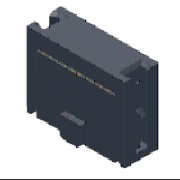
# Autodesk Inventor part: RC CON_16CKT
Saved by Autodesk Inventor 2017 (Build 210142000, 142)
## iProperties
Created: 2016-02-22
Part Number: RC CON_16CKT
Material: Générique
Description: 2,54 mm (0,10 po) Pas, Prise, Vertical, Double ligne
Document SubType Name: Modeling
Designer: Adrien MARY
Language: fr-FR
Size Designation: Ribbon Cable Connector-04
Categories: <MemberInstance><Categories><Category DisplayName="Câble et faisceau" InternalName="e4a7e005-5e42-4d16-b293-125e7f0d0512" Mnemonic="CABLEANDHARNESS"><Category DisplayName="Raccords" InternalName="6f634eba-a678-4820-a31d-2c2d5ee6728e" Mnemonic="CONNECTORS"><CategoryParameter DisplayName="RefDes" InternalName="c3740e8c-60ab-4d5d-8584-52b73222f2f0" Mnemonic="REFDES"/><Category DisplayName="Câble-ruban" InternalName="27621a3d-53ec-49ed-8225-e2ac65e8eb52" Mnemonic="RIBBONCABLE"/></Category></Category><Category DisplayName="Type de données" InternalName="23b78d0f-2648-40c6-8793-ca6db495c9e8" Mnemonic="DATATYPE"><CategoryParameter DisplayName="AfficherNom" InternalName="05415f3d-3907-474b-a020-eb9d644f4cf3" Mnemonic="DISPLAYNAME"/><CategoryParameter DisplayName="Norme" InternalName="0c0a119c-1e12-4c84-803f-101930972f5e" Mnemonic="STANDARD"/><CategoryParameter DisplayName="Description" InternalName="13903e3d-64b1-4950-80da-f627842ea37f" Mnemonic="DESCRIPTION"/><CategoryParameter DisplayName="Désignation" InternalName="2675968c-4ce5-49e0-a4f5-552d29089031" Mnemonic="DESIGNATION"/><CategoryParameter DisplayName="Ligne par défaut" InternalName="2af9ec52-faaa-4026-b378-f9fa4afca842" Mnemonic="DEFAULTROW"/><CategoryParameter DisplayName="Nom de dossier" InternalName="3f06958e-8713-4116-9be7-ed6184ecc97b" Mnemonic="FOLDERNAME"/><CategoryParameter DisplayName="Guide révision" InternalName="45a75005-10b1-4dfc-8d6d-dfe629f0b93c" Mnemonic="REVISIONGUID"/><CategoryParameter DisplayName="NomFichier" InternalName="8b46a4cc-9585-4fed-90c3-899f57e09a73" Mnemonic="FILENAME"/><CategoryParameter DisplayName="OrgNorm" InternalName="8f5914e1-4693-403f-8ab5-d37768198c9d" Mnemonic="STDSORG"/><CategoryParameter DisplayName="Version de la famille" InternalName="914462f6-6e19-4b14-ba84-155b9680b1d0" Mnemonic="FAMILYREVISION"/><CategoryParameter DisplayName="Version standard" InternalName="91d5a463-65c2-4fde-b823-3b7fea5e8e17" Mnemonic="STANDARDREVISION"/><CategoryParameter DisplayName="Révision de membre" InternalName="a65d44b9-392f-4f4f-857b-e4b3d54996fe" Mnemonic="MEMBERREVISION"/><CategoryParameter DisplayName="DélimiterFormat" InternalName="bc51e27b-3422-4e78-93ef-cec197ddf230" Mnemonic="CLIPFORMAT"/><CategoryParameter DisplayName="Fabricant" InternalName="cd6c7a72-a28a-4e50-99a9-2c7f4e13e5ad" Mnemonic="MANUFACTURER"/><CategoryParameter DisplayName="NomInterne" InternalName="cf1d0246-76d9-4b4a-8305-fa0409afb5c1" Mnemonic="INTERNALNAME"/><CategoryParameter DisplayName="Métrique" InternalName="e2385c5b-1ea4-4823-96a8-8de651266ec3" Mnemonic="ISMETRIC"/><Category DisplayName="Pièce" InternalName="c0e0b642-3bcb-4cc8-9e80-f96d35c4afa4" Mnemonic="PART"><CategoryParameter DisplayName="Numéro de pièce" InternalName="016b6077-bfbe-49bd-92c9-d8d59c39c941" Mnemonic="PARTNUMBER"/><CategoryParameter DisplayName="Numéro de stock" InternalName="4dba7c1c-e26c-444e-836c-b08b433409a8" Mnemonic="STOCKNUMBER"/><CategoryParameter DisplayName="Clé matière" InternalName="5c9a8adb-dd2b-4535-b97f-0a94a95fe41f" Mnemonic="MATERIALKEY"/><CategoryParameter DisplayName="Matière" InternalName="818a152a-d3c3-49ca-80ee-df7d91421b8e" Mnemonic="MATERIAL"/></Category></Category></Categories><FamilyTemplate Id="Ribbon Cable Connector"><FamilyTemplateParameters><FamilyTemplateParameter ObjectType="kUserParameterObject" ValueType="xs:double" Id="1" ObjectReferenceKey="Circuits"/><FamilyTemplateParameter ObjectType="kUserParameterObject" ValueType="xs:double" Id="2" ObjectReferenceKey="DimA"/><FamilyTemplateParameter ObjectType="kUserParameterObject" ValueType="xs:double" Id="3" ObjectReferenceKey="DimB"/><FamilyTemplateParameter ObjectType="kPropertyObject" ValueType="xs:string" Id="100" ObjectReferenceKey="{32853F0F-3444-11d1-9E93-0060B03C1CA6}" SubObjectId="52"/><FamilyTemplateParameter ObjectType="kPropertyObject" ValueType="xs:string" Id="105" ObjectReferenceKey="{32853F0F-3444-11d1-9E93-0060B03C1CA6}" SubObjectId="5"/><FamilyTemplateParameter ObjectType="kPartComponentDefinitionObject" ValueType="xs:string" Id="110" SubObjectId="Material"/><FamilyTemplateParameter ObjectType="kPartFeatureObject" ValueType="xs:boolean" Id="200" ObjectReferenceKey="1002000010000000700a0100000000008000000000000000" SubObjectId="Suppressed"/><FamilyTemplateParameter ObjectType="kPartFeatureObject" ValueType="xs:boolean" Id="201" ObjectReferenceKey="1002000010000000320b0100000000008000000000000000" SubObjectId="Suppressed"/><FamilyTemplateParameter ObjectType="kPartFeatureObject" ValueType="xs:boolean" Id="202" ObjectReferenceKey="100200001000000044680200000000008000000000000000" SubObjectId="Suppressed"/><FamilyTemplateParameter ObjectType="kPartFeatureObject" ValueType="xs:boolean" Id="203" ObjectReferenceKey="100200001000000061680200000000008000000000000000" SubObjectId="Suppressed"/><FamilyTemplateParameter ObjectType="kPartFeatureObject" ValueType="xs:boolean" Id="204" ObjectReferenceKey="100200001000000064680200000000008000000000000000" SubObjectId="Suppressed"/><FamilyTemplateParameter ObjectType="kPartFeatureObject" ValueType="xs:boolean" Id="205" ObjectReferenceKey="100200001000000067680200000000008000000000000000" SubObjectId="Suppressed"/><FamilyTemplateParameter ObjectType="kPartFeatureObject" ValueType="xs:boolean" Id="206" ObjectReferenceKey="10020000100000006a680200000000008000000000000000" SubObjectId="Suppressed"/><FamilyTemplateParameter ObjectType="kPartFeatureObject" ValueType="xs:boolean" Id="207" ObjectReferenceKey="10020000100000006d680200000000008000000000000000" SubObjectId="Suppressed"/><FamilyTemplateParameter ObjectType="kPartFeatureObject" ValueType="xs:boolean" Id="208" ObjectReferenceKey="100200001000000070680200000000008000000000000000" SubObjectId="Suppressed"/><FamilyTemplateParameter ObjectType="kPartFeatureObject" ValueType="xs:boolean" Id="209" ObjectReferenceKey="100200001000000073680200000000008000000000000000" SubObjectId="Suppressed"/><FamilyTemplateParameter ObjectType="kPartFeatureObject" ValueType="xs:boolean" Id="210" ObjectReferenceKey="100200001000000076680200000000008000000000000000" SubObjectId="Suppressed"/><FamilyTemplateParameter ObjectType="kPartFeatureObject" ValueType="xs:boolean" Id="211" ObjectReferenceKey="100200001000000079680200000000008000000000000000" SubObjectId="Suppressed"/><FamilyTemplateParameter ObjectType="kPartFeatureObject" ValueType="xs:boolean" Id="212" ObjectReferenceKey="10020000100000007c680200000000008000000000000000" SubObjectId="Suppressed"/><FamilyTemplateParameter ObjectType="kPartFeatureObject" ValueType="xs:boolean" Id="213" ObjectReferenceKey="100200001000000047680200000000008000000000000000" SubObjectId="Suppressed"/><FamilyTemplateParameter ObjectType="kPartFeatureObject" ValueType="xs:boolean" Id="214" ObjectReferenceKey="10020000100000007f680200000000008000000000000000" SubObjectId="Suppressed"/><FamilyTemplateParameter ObjectType="kPartFeatureObject" ValueType="xs:boolean" Id="215" ObjectReferenceKey="100200001000000082680200000000008000000000000000" SubObjectId="Suppressed"/><FamilyTemplateParameter ObjectType="kPartFeatureObject" ValueType="xs:boolean" Id="216" ObjectReferenceKey="100200001000000085680200000000008000000000000000" SubObjectId="Suppressed"/><FamilyTemplateParameter ObjectType="kPartFeatureObject" ValueType="xs:boolean" Id="217" ObjectReferenceKey="100200001000000088680200000000008000000000000000" SubObjectId="Suppressed"/><FamilyTemplateParameter ObjectType="kPartFeatureObject" ValueType="xs:boolean" Id="218" ObjectReferenceKey="10020000100000008b680200000000008000000000000000" SubObjectId="Suppressed"/><FamilyTemplateParameter ObjectType="kPartFeatureObject" ValueType="xs:boolean" Id="219" ObjectReferenceKey="10020000100000008e680200000000008000000000000000" SubObjectId="Suppressed"/><FamilyTemplateParameter ObjectType="kPartFeatureObject" ValueType="xs:boolean" Id="220" ObjectReferenceKey="100200001000000091680200000000008000000000000000" SubObjectId="Suppressed"/><FamilyTemplateParameter ObjectType="kPartFeatureObject" ValueType="xs:boolean" Id="221" ObjectReferenceKey="100200001000000094680200000000008000000000000000" SubObjectId="Suppressed"/><FamilyTemplateParameter ObjectType="kPartFeatureObject" ValueType="xs:boolean" Id="222" ObjectReferenceKey="100200001000000097680200000000008000000000000000" SubObjectId="Suppressed"/><FamilyTemplateParameter ObjectType="kPartFeatureObject" ValueType="xs:boolean" Id="223" ObjectReferenceKey="10020000100000009a680200000000008000000000000000" SubObjectId="Suppressed"/><FamilyTemplateParameter ObjectType="kPartFeatureObject" ValueType="xs:boolean" Id="224" ObjectReferenceKey="10020000100000004a680200000000008000000000000000" SubObjectId="Suppressed"/><FamilyTemplateParameter ObjectType="kPartFeatureObject" ValueType="xs:boolean" Id="225" ObjectReferenceKey="10020000100000009d680200000000008000000000000000" SubObjectId="Suppressed"/><FamilyTemplateParameter ObjectType="kPartFeatureObject" ValueType="xs:boolean" Id="226" ObjectReferenceKey="1002000010000000a0680200000000008000000000000000" SubObjectId="Suppressed"/><FamilyTemplateParameter ObjectType="kPartFeatureObject" ValueType="xs:boolean" Id="227" ObjectReferenceKey="1002000010000000a3680200000000008000000000000000" SubObjectId="Suppressed"/><FamilyTemplateParameter ObjectType="kPartFeatureObject" ValueType="xs:boolean" Id="228" ObjectReferenceKey="1002000010000000a6680200000000008000000000000000" SubObjectId="Suppressed"/><FamilyTemplateParameter ObjectType="kPartFeatureObject" ValueType="xs:boolean" Id="229" ObjectReferenceKey="1002000010000000a9680200000000008000000000000000" SubObjectId="Suppressed"/><FamilyTemplateParameter ObjectType="kPartFeatureObject" ValueType="xs:boolean" Id="230" ObjectReferenceKey="1002000010000000ac680200000000008000000000000000" SubObjectId="Suppressed"/><FamilyTemplateParameter ObjectType="kPartFeatureObject" ValueType="xs:boolean" Id="231" ObjectReferenceKey="1002000010000000af680200000000008000000000000000" SubObjectId="Suppressed"/><FamilyTemplateParameter ObjectType="kPartFeatureObject" ValueType="xs:boolean" Id="232" ObjectReferenceKey="1002000010000000b2680200000000008000000000000000" SubObjectId="Suppressed"/><FamilyTemplateParameter ObjectType="kPartFeatureObject" ValueType="xs:boolean" Id="233" ObjectReferenceKey="1002000010000000b5680200000000008000000000000000" SubObjectId="Suppressed"/><FamilyTemplateParameter ObjectType="kPartFeatureObject" ValueType="xs:boolean" Id="234" ObjectReferenceKey="1002000010000000b8680200000000008000000000000000" SubObjectId="Suppressed"/><FamilyTemplateParameter ObjectType="kPartFeatureObject" ValueType="xs:boolean" Id="235" ObjectReferenceKey="10020000100000004f680200000000008000000000000000" SubObjectId="Suppressed"/><FamilyTemplateParameter ObjectType="kPartFeatureObject" ValueType="xs:boolean" Id="236" ObjectReferenceKey="1002000010000000bb680200000000008000000000000000" SubObjectId="Suppressed"/><FamilyTemplateParameter ObjectType="kPartFeatureObject" ValueType="xs:boolean" Id="237" ObjectReferenceKey="1002000010000000be680200000000008000000000000000" SubObjectId="Suppressed"/><FamilyTemplateParameter ObjectType="kPartFeatureObject" ValueType="xs:boolean" Id="238" ObjectReferenceKey="1002000010000000c1680200000000008000000000000000" SubObjectId="Suppressed"/><FamilyTemplateParameter ObjectType="kPartFeatureObject" ValueType="xs:boolean" Id="239" ObjectReferenceKey="1002000010000000c4680200000000008000000000000000" SubObjectId="Suppressed"/><FamilyTemplateParameter ObjectType="kPartFeatureObject" ValueType="xs:boolean" Id="240" ObjectReferenceKey="1002000010000000c7680200000000008000000000000000" SubObjectId="Suppressed"/><FamilyTemplateParameter ObjectType="kPartFeatureObject" ValueType="xs:boolean" Id="241" ObjectReferenceKey="1002000010000000ca680200000000008000000000000000" SubObjectId="Suppressed"/><FamilyTemplateParameter ObjectType="kPartFeatureObject" ValueType="xs:boolean" Id="242" ObjectReferenceKey="1002000010000000cd680200000000008000000000000000" SubObjectId="Suppressed"/><FamilyTemplateParameter ObjectType="kPartFeatureObject" ValueType="xs:boolean" Id="243" ObjectReferenceKey="1002000010000000d0680200000000008000000000000000" SubObjectId="Suppressed"/><FamilyTemplateParameter ObjectType="kPartFeatureObject" ValueType="xs:boolean" Id="244" ObjectReferenceKey="1002000010000000d3680200000000008000000000000000" SubObjectId="Suppressed"/><FamilyTemplateParameter ObjectType="kPartFeatureObject" ValueType="xs:boolean" Id="245" ObjectReferenceKey="1002000010000000d6680200000000008000000000000000" SubObjectId="Suppressed"/><FamilyTemplateParameter ObjectType="kPartFeatureObject" ValueType="xs:boolean" Id="246" ObjectReferenceKey="100200001000000052680200000000008000000000000000" SubObjectId="Suppressed"/><FamilyTemplateParameter ObjectType="kPartFeatureObject" ValueType="xs:boolean" Id="247" ObjectReferenceKey="1002000010000000d9680200000000008000000000000000" SubObjectId="Suppressed"/><FamilyTemplateParameter ObjectType="kPartFeatureObject" ValueType="xs:boolean" Id="248" ObjectReferenceKey="1002000010000000dc680200000000008000000000000000" SubObjectId="Suppressed"/><FamilyTemplateParameter ObjectType="kPartFeatureObject" ValueType="xs:boolean" Id="249" ObjectReferenceKey="1002000010000000df680200000000008000000000000000" SubObjectId="Suppressed"/><FamilyTemplateParameter ObjectType="kPartFeatureObject" ValueType="xs:boolean" Id="250" ObjectReferenceKey="1002000010000000e2680200000000008000000000000000" SubObjectId="Suppressed"/><FamilyTemplateParameter ObjectType="kPartFeatureObject" ValueType="xs:boolean" Id="251" ObjectReferenceKey="1002000010000000e5680200000000008000000000000000" SubObjectId="Suppressed"/><FamilyTemplateParameter ObjectType="kPartFeatureObject" ValueType="xs:boolean" Id="252" ObjectReferenceKey="1002000010000000e8680200000000008000000000000000" SubObjectId="Suppressed"/><FamilyTemplateParameter ObjectType="kPartFeatureObject" ValueType="xs:boolean" Id="253" ObjectReferenceKey="1002000010000000eb680200000000008000000000000000" SubObjectId="Suppressed"/><FamilyTemplateParameter ObjectType="kPartFeatureObject" ValueType="xs:boolean" Id="254" ObjectReferenceKey="1002000010000000ee680200000000008000000000000000" SubObjectId="Suppressed"/><FamilyTemplateParameter ObjectType="kPartFeatureObject" ValueType="xs:boolean" Id="255" ObjectReferenceKey="1002000010000000f1680200000000008000000000000000" SubObjectId="Suppressed"/><FamilyTemplateParameter ObjectType="kPartFeatureObject" ValueType="xs:boolean" Id="256" ObjectReferenceKey="1002000010000000f4680200000000008000000000000000" SubObjectId="Suppressed"/><FamilyTemplateParameter ObjectType="kPartFeatureObject" ValueType="xs:boolean" Id="257" ObjectReferenceKey="100200001000000055680200000000008000000000000000" SubObjectId="Suppressed"/><FamilyTemplateParameter ObjectType="kPartFeatureObject" ValueType="xs:boolean" Id="258" ObjectReferenceKey="1002000010000000f7680200000000008000000000000000" SubObjectId="Suppressed"/><FamilyTemplateParameter ObjectType="kPartFeatureObject" ValueType="xs:boolean" Id="259" ObjectReferenceKey="1002000010000000fa680200000000008000000000000000" SubObjectId="Suppressed"/><FamilyTemplateParameter ObjectType="kPartFeatureObject" ValueType="xs:boolean" Id="260" ObjectReferenceKey="1002000010000000fd680200000000008000000000000000" SubObjectId="Suppressed"/><FamilyTemplateParameter ObjectType="kPartFeatureObject" ValueType="xs:boolean" Id="261" ObjectReferenceKey="100200001000000000690200000000008000000000000000" SubObjectId="Suppressed"/><FamilyTemplateParameter ObjectType="kPartFeatureObject" ValueType="xs:boolean" Id="262" ObjectReferenceKey="100200001000000003690200000000008000000000000000" SubObjectId="Suppressed"/><FamilyTemplateParameter ObjectType="kPartFeatureObject" ValueType="xs:boolean" Id="263" ObjectReferenceKey="100200001000000058680200000000008000000000000000" SubObjectId="Suppressed"/><FamilyTemplateParameter ObjectType="kPartFeatureObject" ValueType="xs:boolean" Id="264" ObjectReferenceKey="10020000100000005b680200000000008000000000000000" SubObjectId="Suppressed"/><FamilyTemplateParameter ObjectType="kPartFeatureObject" ValueType="xs:boolean" Id="265" ObjectReferenceKey="10020000100000005e680200000000008000000000000000" SubObjectId="Suppressed"/></FamilyTemplateParameters></FamilyTemplate><CategoryParameterMap><ParamToTemplateMap><ParamToTemplate CategoryParameter="//CategoryParameter[@InternalName='05415f3d-3907-474b-a020-eb9d644f4cf3']" ConstantValue="Ribbon Cable Connector"/><ParamToTemplate CategoryParameter="//CategoryParameter[@InternalName='0c0a119c-1e12-4c84-803f-101930972f5e']" TemplateParameter="102"/><ParamToTemplate CategoryParameter="//CategoryParameter[@InternalName='13903e3d-64b1-4950-80da-f627842ea37f']" ConstantValue="2.54mm (0.10in) Pitch, Receptacle, Vertical, Dual Row"/><ParamToTemplate CategoryParameter="//CategoryParameter[@InternalName='2af9ec52-faaa-4026-b378-f9fa4afca842']" ConstantValue="1"/><ParamToTemplate CategoryParameter="//CategoryParameter[@InternalName='3f06958e-8713-4116-9be7-ed6184ecc97b']" ConstantValue="Ribbon Cable Connector"/><ParamToTemplate CategoryParameter="//CategoryParameter[@InternalName='45a75005-10b1-4dfc-8d6d-dfe629f0b93c']" ConstantValue="a3a57e36-970e-4b53-b58b-44e930e7e04d"/><ParamToTemplate CategoryParameter="//CategoryParameter[@InternalName='8f5914e1-4693-403f-8ab5-d37768198c9d']" TemplateParameter="101"/><ParamToTemplate CategoryParameter="//CategoryParameter[@InternalName='914462f6-6e19-4b14-ba84-155b9680b1d0']" ConstantValue="11"/><ParamToTemplate CategoryParameter="//CategoryParameter[@InternalName='91d5a463-65c2-4fde-b823-3b7fea5e8e17']" TemplateParameter="103"/><ParamToTemplate CategoryParameter="//CategoryParameter[@InternalName='bc51e27b-3422-4e78-93ef-cec197ddf230']" ConstantValue="CF_INVENTOR.STDPARTS"/><ParamToTemplate CategoryParameter="//CategoryParameter[@InternalName='cd6c7a72-a28a-4e50-99a9-2c7f4e13e5ad']" TemplateParameter="104"/><ParamToTemplate CategoryParameter="//CategoryParameter[@InternalName='cf1d0246-76d9-4b4a-8305-fa0409afb5c1']" ConstantValue="40b76d18-17cd-4eeb-a7c8-2b6dc5bd681a"/><ParamToTemplate CategoryParameter="//CategoryParameter[@InternalName='e2385c5b-1ea4-4823-96a8-8de651266ec3']" ConstantValue="true"/><ParamToTemplate CategoryParameter="//CategoryParameter[@InternalName='8b46a4cc-9585-4fed-90c3-899f57e09a73']" ConstantValue="Ribbon Cable Connector-04"/><ParamToTemplate CategoryParameter="//CategoryParameter[@InternalName='a65d44b9-392f-4f4f-857b-e4b3d54996fe']" ConstantValue="b666cb32-0b43-4429-87d9-31e43f82d377"/><ParamToTemplate CategoryParameter="//CategoryParameter[@InternalName='2675968c-4ce5-49e0-a4f5-552d29089031']" TemplateParameter="100"/><ParamToTemplate CategoryParameter="//CategoryParameter[@InternalName='818a152a-d3c3-49ca-80ee-df7d91421b8e']" TemplateParameter="110"/><ParamToTemplate CategoryParameter="//CategoryParameter[@InternalName='016b6077-bfbe-49bd-92c9-d8d59c39c941']" TemplateParameter="105"/></ParamToTemplateMap></CategoryParameterMap></MemberInstance>
Density: 1 g/cm^3
Appearance: Dark Gray
IsCustomPart: 0
Author: Adrien MARY
Autodesk Inventor part; units mm, degrees
ref_plane "YZ Plane" through (0, 0, 0) normal (1, 0, 0) x (0, 1, 0)
ref_plane "XZ Plane" through (0, 0, 0) normal (0, 1, 0) x (-1, 0, 0)
ref_plane "XY Plane" through (0, 0, 0) normal (0, 0, 1) x (1, 0, 0)
sketch "Sketch1" plane through (0, 0, 0) normal (0, 0, 1) x (1, 0, 0)
  line L0 (10.79, -3) -> (-10.79, -3)
  line L1 (-10.79, -1.5) -> (-10.04, -1.5)
  line L2 (-10.04, -1.5) -> (-10.04, -2.1)
  line L3 (-10.04, -2.1) -> (-10.79, -2.1)
  line L4 (-10.79, -3) -> (-10.79, -2.1)
  line L5 (-10.79, -1.5) -> (-10.79, 3)
  line L6 (10.04, 2.1) -> (10.79, 2.1)
  line L7 (10.79, 1.5) -> (10.04, 1.5)
  line L8 (10.04, 1.5) -> (10.04, 2.1)
  line L9 (10.79, 3) -> (10.79, 2.1)
  line L10 (10.79, 1.5) -> (10.79, -3)
  line L11 (0, 3) -> (0, -3) construction
  line L12 (-10.79, 3) -> (10.79, 3)
  point P0 (0, 0)
  point P1 (0, 0)
  dimension "d0" = 21.58
  dimension "d1" = 6
  dimension "d4" = 0.9
  dimension "d5" = 0.75
  dimension "d6" = 0.6
  dimension "d8" = 0.75
  dimension "d9" = 0.6
  dimension "d10" = 6
  dimension "d12" = 0.9
  constraints: 26 end point, 8 parallel, 3 midpoint, 3 perpendicular, 2 horizontal, 1 coincident
  measures "d0" distance of L0.start L0.end
  measures "d1" distance of L0.end L5.end
  measures "d4" distance between parallel lines of L0 L3
  measures "d5" distance of L2.end L4.end
  measures "d6" distance of L2.start L2.end
  measures "d8" distance of L8.end L6.end
  measures "d9" distance of L8.start L8.end
  measures "d10" distance of L0.start L9.start
  measures "d12" distance of L9.start L6.end
extrude "Extrusion1" add sketch "Sketch1" along normal blind 10.2
sketch "Sketch2" plane through (-10.79, -3, 0) normal (0, -1, 0) x (1, 0, 0)
  line L0 (0, 0) -> (21.58, 0) projected
  line L1 (8.99, 3.6) -> (12.59, 3.6)
  line L2 (12.59, 3.6) -> (12.59, 0.5)
  line L3 (12.09, 0) -> (9.49, 0)
  line L4 (8.99, 0.5) -> (8.99, 3.6)
  line L5 (8.99, 0.5) -> (9.49, 0)
  line L6 (12.59, 0.5) -> (12.09, 0)
  point P0 (10.79, 0)
  dimension "d15" = 3.6
  dimension "d17" = 0.5
  dimension "d19" = 135
  dimension "d20" = 135
  dimension "d21" = 0.5
  dimension "d22" = 3.6
  constraints: 12 end point, 2 midpoint, 2 parallel, 1 horizontal, 1 perpendicular
  measures "d15" distance of L1.start L1.end
  measures "d17" horizontal distance of L3.end L4.start
  measures "d19" angle of L5 L4
  measures "d20" angle of L6 L2
  measures "d21" horizontal distance of L3.start L2.end
  measures "d22" distance between parallel lines of L0 L1
extrude "Extrusion2" add sketch "Sketch2" along normal blind 1
sketch "Sketch3" plane through (0, 0, 0) normal (0, 1, 0) x (-1, 0, 0)
  line L0 (-10.79, 3.6) -> (-11.04, 3.6)
  line L1 (-11.79, 2.1) -> (-11.79, 1.22)
  line L2 (-11.79, 1.22) -> (-10.79, 1.22)
  line L3 (-10.79, 1.22) -> (-10.79, 3.6)
  line L4 (10.79, 10.2) -> (-10.79, 10.2) projected
  line L5 (0, 10.2) -> (0, 0)
  line L6 (-10.79, 0) -> (10.79, 0) projected
  line L7 (-11.04, 3.6) -> (-11.79, 2.1)
  line L8 (10.79, 3.6) -> (11.04, 3.6)
  line L9 (11.79, 2.1) -> (11.79, 1.22)
  line L10 (11.79, 1.22) -> (10.79, 1.22)
  line L11 (10.79, 1.22) -> (10.79, 3.6)
  line L12 (11.04, 3.6) -> (11.79, 2.1)
  dimension "d25" = 21.58
  dimension "d26" = 1.22
  dimension "d28" = 1
  dimension "d29" = 1.5
  dimension "d30" = 0.88
  dimension "d31" = 0.25
  constraints: 22 end point, 5 symmetric about line, 2 midpoint, 2 parallel, 2 perpendicular, 1 horizontal
  measures "d25" diameter of L3 L5
  measures "d26" distance between parallel lines of L2 L6
  measures "d28" distance of L1.end L2.end
  measures "d29" vertical distance of L0.end L1.start
  measures "d30" distance of L1.start L1.end
  measures "d31" distance of L0.start L0.end
extrude "Extrusion3" add sketch "Sketch3" along normal mid plane 1
sketch "Sketch4" plane through (0, -0.5, 0) normal (0, -1, 0) x (1, 0, 0)
  line L0 (10.79, 3.6) -> (11.04, 3.6) projected
  line L1 (10.79, 6.263) -> (11.04, 6.263)
  line L2 (11.79, 5.513) -> (11.79, 5.263)
  line L3 (11.79, 5.263) -> (10.79, 5.263)
  line L4 (10.79, 5.263) -> (10.79, 6.263)
  line L5 (-10.79, 10.2) -> (10.79, 10.2) projected
  line L6 (10.79, 0) -> (-10.79, 0) projected
  line L7 (0, 10.2) -> (0, 0)
  line L8 (11.04, 6.263) -> (11.79, 5.513)
  line L9 (-10.79, 6.263) -> (-11.04, 6.263)
  line L10 (-11.79, 5.513) -> (-11.79, 5.263)
  line L11 (-11.79, 5.263) -> (-10.79, 5.263)
  line L12 (-10.79, 5.263) -> (-10.79, 6.263)
  line L13 (-11.04, 6.263) -> (-11.79, 5.513)
  dimension "d34" = 1.663
  dimension "d35" = 21.58
  dimension "d36" = 1
  dimension "d38" = 0.25
  dimension "d39" = 1
  dimension "d40" = 0.25
  constraints: 22 end point, 5 symmetric about line, 2 midpoint, 2 parallel, 1 horizontal, 1 perpendicular
  measures "d34" distance between parallel lines of L3 L0
  measures "d35" diameter of L4 L7
  measures "d36" distance of L2.end L3.end
  measures "d38" distance of L1.start L1.end
  measures "d39" distance of L3.end L1.start
  measures "d40" distance of L2.start L2.end
extrude "Extrusion4" add sketch "Sketch4" along normal blind 1
sketch "Sketch5" plane through (0, 0.5, 0) normal (0, 1, 0) x (1, 0, 0)
  line L0 (11.04, -3.6) -> (10.79, -3.6) projected
  line L1 (11.04, -6.263) -> (10.79, -6.263)
  line L2 (10.79, -6.263) -> (10.79, -5.263)
  line L3 (10.79, -5.263) -> (11.79, -5.263)
  line L4 (11.79, -5.263) -> (11.79, -5.513)
  line L5 (10.79, -10.2) -> (-10.79, -10.2) projected
  line L6 (1.3, 0) -> (-1.3, 0) projected
  line L7 (0, 0) -> (0, -10.2)
  line L8 (11.04, -6.263) -> (11.79, -5.513)
  line L9 (-11.04, -6.263) -> (-10.79, -6.263)
  line L10 (-10.79, -6.263) -> (-10.79, -5.263)
  line L11 (-10.79, -5.263) -> (-11.79, -5.263)
  line L12 (-11.79, -5.263) -> (-11.79, -5.513)
  line L13 (-11.04, -6.263) -> (-11.79, -5.513)
  dimension "d43" = 1.663
  dimension "d44" = 21.58
  dimension "d45" = 1
  dimension "d46" = 1
  dimension "d47" = 0.25
  dimension "d48" = 0.25
  constraints: 22 end point, 5 symmetric about line, 2 midpoint, 2 parallel, 1 horizontal, 1 perpendicular
  measures "d43" distance between parallel lines of L0 L3
  measures "d44" diameter of L2 L7
  measures "d45" distance of L1.end L2.end
  measures "d46" distance of L2.end L3.end
  measures "d47" distance of L1.start L1.end
  measures "d48" distance of L3.end L4.end
extrude "Extrusion5" add sketch "Sketch5" along normal blind 1
sketch "Sketch6" plane through (-10.79, -3, 10.2) normal (0, -1, 0) x (1, 0, 0)
  line L0 (0, -10.2) -> (9.49, -10.2) projected
  line L1 (-38.97, -10.2) -> (-36.97, -6.7359)
  line L2 (-36.97, -6.7359) -> (-34.97, -10.2)
  line L3 (-38.97, -10.2) -> (-34.97, -10.2)
  line L4 (0.5, -10.2) -> (2.5, -6.7359)
  line L5 (2.5, -6.7359) -> (4.5, -10.2)
  line L6 (0.5, -10.2) -> (4.5, -10.2)
  dimension "d61" = 0.5
  dimension "d62" = 4
  constraints: 12 end point, 4 equal length, 2 point on line, 1 collinear
  measures "d61" distance of L4.start L0.start
  measures "d62" distance of L4.start L5.end
extrude "Extrusion6" cut sketch "Sketch6" against normal blind 0.1 contours L4 L5 L0
sketch "Sketch7" plane through (0, 0, 0) normal (0, 0, -1) x (-1, 0, 0)
  line L0 (10.79, 3) -> (10.79, -1.5) projected
  line L1 (8.515, 1.645) -> (9.265, 1.645)
  line L2 (9.265, 1.645) -> (9.265, 0.895)
  line L3 (9.265, 0.895) -> (8.515, 0.895)
  line L4 (8.515, 0.895) -> (8.515, 1.645)
  line L5 (8.515, -0.895) -> (9.265, -0.895)
  line L6 (9.265, -0.895) -> (9.265, -1.645)
  line L7 (9.265, -1.645) -> (8.515, -1.645)
  line L8 (8.515, -1.645) -> (8.515, -0.895)
  line L9 (8.89, 0.895) -> (8.89, -0.895) construction
  point P0 (0, 0)
  point P1 (8.89, 0)
  dimension "d65" = 0.75
  dimension "d66" = 2.54
  dimension "d67" = 1.525
  constraints: 18 end point, 7 equal length, 4 parallel, 3 midpoint, 3 perpendicular, 2 horizontal, 1 horizontal alignment
  measures "d65" distance of L1.start L1.end
  measures "d66" distance between parallel lines of L5 L1
  measures "d67" distance between parallel lines of L0 L6
extrude "Extrusion7" cut sketch "Sketch7" against normal blind 3
chamfer "Chanfrein1" distance 0.5 angle 45 8 edges at (-8.89, -1.645, 0) (-8.515, -1.27, 0) (-8.89, -0.895, 0) (-9.265, -1.27, 0) (-8.89, 0.895, 0) (-8.515, 1.27, 0) (-8.89, 1.645, 0) (-9.265, 1.27, 0)
pattern_linear "Réseau rectangulaire1" count 8 spacing 2.54 along (1, 0, 0) of "Extrusion7", "Chanfrein1"
ref_plane "Work Plane1" through (0, 0, 10.7) normal (0, 0, 1) x (1, 0, 0)
sketch "Sketch8" plane through (0, 0, 10.7) normal (0, 0, 1) x (1, 0, 0)
  line L0 (-12.475, 3.03) -> (12.475, 3.03)
  line L1 (12.475, -3.03) -> (-12.475, -3.03)
  line L2 (-12.475, -1.03) -> (-11.7708, -1.4995)
  line L3 (-11.7708, -1.4995) -> (-10.92, -1.4995)
  line L4 (-10.92, -1.4995) -> (-10.92, 1.4995)
  line L5 (-12.475, -3.03) -> (-12.475, -1.03)
  line L6 (-10.79, 3) -> (10.79, 3) projected
  line L7 (-10.79, -1.5) -> (-10.79, 3) projected
  line L8 (-10.04, -1.5) -> (-10.79, -1.5) projected
  line L9 (-10.04, -2.1) -> (-10.04, -1.5) projected
  line L10 (-10.79, -2.1) -> (-10.04, -2.1) projected
  line L11 (-10.79, -3) -> (-10.79, -2.1) projected
  line L12 (10.79, -3) -> (-10.79, -3) projected
  line L13 (10.79, 1.5) -> (10.79, -3) projected
  line L14 (10.04, 1.5) -> (10.79, 1.5) projected
  line L15 (10.04, 2.1) -> (10.04, 1.5) projected
  line L16 (10.79, 2.1) -> (10.04, 2.1) projected
  line L17 (10.79, 3) -> (10.79, 2.1) projected
  line L18 (0, 3) -> (0, -3)
  line L19 (-10.92, 0) -> (-42.9538, 0)
  line L20 (-11.7708, 1.4995) -> (-10.92, 1.4995)
  line L21 (-12.475, 1.03) -> (-11.7708, 1.4995)
  line L22 (-12.475, 3.03) -> (-12.475, 1.03)
  line L23 (11.7708, -1.4995) -> (10.92, -1.4995)
  line L24 (12.475, -1.03) -> (11.7708, -1.4995)
  line L25 (12.475, -3.03) -> (12.475, -1.03)
  line L26 (10.92, -1.4995) -> (10.92, 1.4995)
  line L27 (12.475, 1.03) -> (11.7708, 1.4995)
  line L28 (12.475, 3.03) -> (12.475, 1.03)
  line L29 (11.7708, 1.4995) -> (10.92, 1.4995)
  point P0 (0, 0)
  point P1 (0, 0)
  point P2 (-12.475, -2.03)
  point P3 (0, 0)
  dimension "d160" = 2
  dimension "d161" = 0.8508
  dimension "d162" = 2.9989
  dimension "d163" = 56.31
  dimension "d164" = 0.13
  dimension "d165" = 24.95
  constraints: 36 end point, 8 symmetric about line, 5 midpoint, 4 perpendicular, 3 parallel, 1 coincident, 1 horizontal, 1 horizontal alignment
  measures "d160" distance of L5.start L2.start
  measures "d161" distance of L3.start L3.end
  measures "d162" distance of L3.end L4.end
  measures "d163" angle of L5 L2
  measures "d164" distance between parallel lines of L7 L4
  measures "d165" distance of L0.start L0.end
extrude "Extrusion8" add sketch "Sketch8" along normal blind 2.5 contours L0 L28 L27 L29 L26 L23 L24 L25 L1 L5 L2 L3 L4 L20 L21 L22 | L6 L18 L12 L11 L10 L9 L8 L7 | L6 L17 L16 L15 L14 L13 L12 L18
sketch "Sketch10" plane through (0, 0, 10.7) normal (0, 0, -1) x (-1, 0, 0)
  line L0 (-12.475, 3.03) -> (-12.475, 1.03) projected
  line L1 (12.475, 3.03) -> (-12.475, 3.03) projected
  line L2 (12.475, 1.03) -> (12.475, 3.03) projected
  line L3 (11.7708, 1.4995) -> (12.475, 1.03) projected
  line L4 (10.92, 1.4995) -> (11.7708, 1.4995) projected
  line L5 (10.92, -1.4995) -> (10.92, 1.4995) projected
  line L6 (11.7708, -1.4995) -> (10.92, -1.4995) projected
  line L7 (12.475, -1.03) -> (11.7708, -1.4995) projected
  line L8 (12.475, -3.03) -> (12.475, -1.03) projected
  line L9 (-12.475, -3.03) -> (12.475, -3.03) projected
  line L10 (-12.475, -1.03) -> (-12.475, -3.03) projected
  line L11 (-11.7708, -1.4995) -> (-12.475, -1.03) projected
  line L12 (-10.92, -1.4995) -> (-11.7708, -1.4995) projected
  line L13 (-10.92, 1.4995) -> (-10.92, -1.4995) projected
  line L14 (-11.7708, 1.4995) -> (-10.92, 1.4995) projected
  line L15 (-12.475, 1.03) -> (-11.7708, 1.4995) projected
  line L16 (10.79, -1.5) -> (10.04, -1.5) projected
  line L17 (10.04, -1.5) -> (10.04, -2.1) projected
  line L18 (10.04, -2.1) -> (10.79, -2.1) projected
  line L19 (-10.79, 1.5) -> (-10.04, 1.5) projected
  line L20 (-10.04, 1.5) -> (-10.04, 2.1) projected
  line L21 (-10.04, 2.1) -> (-10.79, 2.1) projected
  line L22 (-10.8, 1.51) -> (-10.05, 1.51)
  line L23 (-10.05, 1.51) -> (-10.05, 2.09)
  line L24 (-10.05, 2.09) -> (-10.8, 2.09)
  line L25 (-10.8, 2.09) -> (-10.8, 3.03)
  line L26 (10.8, -2.09) -> (10.05, -2.09)
  line L27 (10.05, -2.09) -> (10.05, -1.51)
  line L28 (10.05, -1.51) -> (10.8, -1.51)
  line L29 (10.8, -3.03) -> (10.8, -2.09)
  line L30 (-10.92, -1.4995) -> (-10.8, -1.4995)
  line L31 (-10.92, 1.4995) -> (-10.8, 1.4995)
  line L32 (-10.8, -3.03) -> (-10.8, -1.4995)
  line L33 (-10.8, 1.4995) -> (-10.8, 1.51)
  line L34 (10.92, 1.4995) -> (10.8, 1.4995)
  line L35 (10.92, -1.4995) -> (10.8, -1.4995)
  line L36 (10.8, -1.51) -> (10.8, -1.4995)
  line L37 (10.8, 1.4995) -> (10.8, 3.03)
  point P0 (-10.05, 1.8)
  point P1 (-10.04, 1.8)
  point P2 (10.05, -1.8)
  point P3 (10.04, -1.8)
  dimension "d167" = 0.01
  dimension "d168" = 0.01
  dimension "d170" = 0.01
  dimension "d172" = 0.01
  dimension "d173" = 0.01
  dimension "d174" = 0.01
  dimension "d180" = 0.01
  dimension "d181" = 0.12
  dimension "d182" = 0.01
  dimension "d183" = 0.12
  constraints: 32 end point, 8 perpendicular, 7 parallel, 4 midpoint, 4 point on line, 2 horizontal, 2 horizontal alignment
  measures "d167" distance between parallel lines of L19 L22
  measures "d168" distance between parallel lines of L20 L23
  measures "d170" distance from line of L25 L21.end
  measures "d172" distance between parallel lines of L18 L26
  measures "d173" distance between parallel lines of L17 L27
  measures "d174" distance from line of L29 L18.end
  measures "d180" distance from line of L19.start L33
  measures "d181" distance of L12.start L30.end
  measures "d182" distance of L35.end L16.start
  measures "d183" distance of L4.start L34.end
extrude "Extrusion9" add sketch "Sketch10" along normal blind 10.7 contours L1 L25 L24 L23 L22 L33 L31 L14 L15 L0 | L1 L2 L3 L4 L34 L37 | L30 L32 L9 L10 L11 L12 | L6 L7 L8 L9 L29 L26 L27 L28 L36 L35
sketch "Sketch12" plane through (0, 0, 0) normal (0, 1, 0) x (-1, 0, 0)
  line L0 (12.475, 13.2) -> (-12.475, 13.2) projected
  line L1 (0, 13.2) -> (0, 4.8655)
  line L2 (-12.475, 13.2) -> (-12.475, 0) projected
  line L3 (-12.475, 0) -> (-10.8, 0)
  line L4 (-10.8, 0) -> (-10.8, 1.21)
  line L5 (-10.8, 1.21) -> (-12.475, 1.21)
  line L6 (-12.475, 1.21) -> (-12.475, 0)
  line L7 (-11.04, 3.6) -> (-10.79, 3.6) projected
  line L8 (-11.79, 2.1) -> (-11.04, 3.6) projected
  line L9 (-11.79, 1.22) -> (-11.79, 2.1) projected
  line L10 (-10.79, 1.22) -> (-11.79, 1.22) projected
  line L11 (12.475, 0) -> (10.8, 0)
  line L12 (10.8, 0) -> (10.8, 1.21)
  line L13 (10.8, 1.21) -> (12.475, 1.21)
  line L14 (12.475, 1.21) -> (12.475, 0)
  line L15 (-10.79, 3.6) -> (-10.79, 1.22) projected
  dimension "d177" = 0.01
  dimension "d243" = 1.675
  constraints: 18 end point, 4 symmetric about line, 2 parallel, 2 perpendicular, 1 horizontal, 1 midpoint
  measures "d177" distance between parallel lines of L10 L5
  measures "d243" distance of L2.end L3.end
extrude "Extrusion10" add sketch "Sketch12" along normal mid plane 6.06 contours L5 L4 L3 L2 | L11 L12 L13 L14
chamfer "Chanfrein2" distance 1 angle 45 4 edges at (10.8, -0.76, 0) (10.8, 2.56, 0) (-10.8, -2.56, 0) (-10.8, 0.76, 0)
chamfer "Chanfrein3" distance 1.749 angle 45 2 edges at (-10.05, -1.8, 0) (10.05, 1.8, 0)
chamfer "Chanfrein4" distance 10.71 distance2 0.03 1 edges at (12.1375, -3.03, 0) measured on face at (12.1375, -3.03, 0.5)
chamfer "Chanfrein5" distance 10.71 distance2 0.03 1 edges at (12.1375, 3.03, 0) measured on face at (12.1375, 3.03, 0.5)
chamfer "Chanfrein8" distance 0.5 angle 45 10 edges at (10.92, 0, 13.2) (11.3454, 1.4995, 13.2) (12.1229, 1.2647, 13.2) (11.3454, -1.4995, 13.2) (12.1229, -1.2647, 13.2) (-12.1229, 1.2647, 13.2) (-11.3454, 1.4995, 13.2) (-10.92, 0, 13.2) (-11.3454, -1.4995, 13.2) (-12.1229, -1.2647, 13.2)
sketch "Sketch20" plane through (-12.475, -3.03, 13.2) normal (0, -1, 0) x (1, 0, 0)
  line L0 (24.95, -2.49) -> (0, -2.49) projected
  line L1 (24.95, 0) -> (24.95, -2.49) projected
  line L2 (24.95, 0) -> (0, 0) projected
  line L3 (0, 0) -> (0, -2.49) projected
  line L4 (23.265, -3) -> (1.685, -3) projected
  point P0 (2.95, -2.75)
  point P1 (12.475, -2.75)
  point P2 (12.475, 0.25)
  point P3 (12.475, -2.49)
  point P4 (12.475, 0)
  point P5 (4.22, -2.75)
  point P6 (5.49, -2.75)
  point P7 (6.76, -2.75)
  point P8 (8.03, -2.75)
  point P9 (9.3, -2.75)
  point P10 (10.57, -2.75)
  point P11 (11.84, -2.75)
  point P12 (13.11, -2.75)
  point P13 (14.38, -2.75)
  point P14 (15.65, -2.75)
  point P15 (16.92, -2.75)
  point P16 (18.19, -2.75)
  point P17 (19.46, -2.75)
  point P18 (20.73, -2.75)
  point P19 (22, -2.75)
  point P20 (23.27, -2.75)
  point P21 (24.54, -2.75)
  point P22 (25.81, -2.75)
  point P23 (27.08, -2.75)
  point P24 (28.35, -2.75)
  point P25 (29.62, -2.75)
  point P26 (30.89, -2.75)
  point P27 (32.16, -2.75)
  point P28 (33.43, -2.75)
  point P29 (34.7, -2.75)
  point P30 (35.97, -2.75)
  point P31 (37.24, -2.75)
  point P32 (38.51, -2.75)
  point P33 (39.78, -2.75)
  point P34 (41.05, -2.75)
  point P35 (42.32, -2.75)
  point P36 (43.59, -2.75)
  point P37 (44.86, -2.75)
  point P38 (46.13, -2.75)
  point P39 (47.4, -2.75)
  point P40 (48.67, -2.75)
  point P41 (49.94, -2.75)
  point P42 (51.21, -2.75)
  point P43 (52.48, -2.75)
  point P44 (53.75, -2.75)
  point P45 (55.02, -2.75)
  point P46 (56.29, -2.75)
  point P47 (57.56, -2.75)
  point P48 (58.83, -2.75)
  point P49 (60.1, -2.75)
  point P50 (61.37, -2.75)
  point P51 (62.64, -2.75)
  point P52 (63.91, -2.75)
  point P53 (65.18, -2.75)
  point P54 (66.45, -2.75)
  point P55 (67.72, -2.75)
  point P56 (68.99, -2.75)
  point P57 (70.26, -2.75)
  point P58 (71.53, -2.75)
  point P59 (72.8, -2.75)
  point P60 (74.07, -2.75)
  point P61 (75.34, -2.75)
  point P62 (76.61, -2.75)
  point P63 (77.88, -2.75)
  point P64 (79.15, -2.75)
  point P65 (80.42, -2.75)
  point P66 (81.69, -2.75)
  point P67 (82.96, -2.75)
  dimension "d240" = 0.25
  dimension "d241" = 0.25
  dimension "d242" = 0.25
  dimension "d247" = 9.525
  dimension "d250" = 1.27
  constraints: 2 midpoint, 2 vertical alignment, 1 horizontal, 63 other
  measures "d240" distance from line of L4 point (2.95, -2.75)
  measures "d241" distance from line of L4 point (12.475, -2.75)
  measures "d242" distance from line of L2 point (12.475, 0.25)
  measures "d247" distance of point (12.475, -2.75) point (2.95, -2.75)
  measures "d250" distance of point (2.95, -2.75) point (4.22, -2.75)
sketch "Sketch21" plane through (-12.475, 3.03, 13.2) normal (0, 1, 0) x (1, 0, 0)
  line L0 (0, 2.49) -> (24.95, 2.49) projected
  line L1 (0, 2.49) -> (0, 0) projected
  line L2 (0, 0) -> (24.95, 0) projected
  line L3 (24.95, 0) -> (24.95, 2.49) projected
  point P0 (12.475, -0.25)
  point P1 (12.475, 2.75)
equation "\"DimA\" = 21.58"
equation "\"DimB\" = 24.95"
equation "\"DimC\" = 9.525"
body "Solid1"
